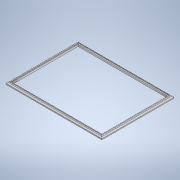
# Autodesk Inventor part: Square
Saved by Autodesk Inventor 2021 (Build 250183000, 183)
## iProperties
Created: 2022-03-13
Part Number: Square
Material: Generic
Document SubType Name: Modeling
Designer: stefi
Density: 1 g/cm^3
Appearance: Default
Author: stefi
Autodesk Inventor part; units mm, degrees
ref_plane "YZ Plane" through (0, 0, 0) normal (1, 0, 0) x (0, 1, 0)
ref_plane "XZ Plane" through (0, 0, 0) normal (0, 1, 0) x (-1, 0, 0)
ref_plane "XY Plane" through (0, 0, 0) normal (0, 0, 1) x (1, 0, 0)
sketch "Sketch2" plane through (0, 0, 0) normal (0, 1, 0) x (-1, 0, 0)
  line L0 (357.886, 268.986) -> (-357.886, 268.986)
  line L1 (-357.886, 268.986) -> (-357.886, -268.986)
  line L2 (-357.886, -268.986) -> (357.886, -268.986)
  line L3 (357.886, -268.986) -> (357.886, 268.986)
  line L4 (357.886, 268.986) -> (-357.886, -268.986) construction
  line L5 (-357.886, 268.986) -> (357.886, -268.986) construction
  line L6 (334.899, 245.999) -> (-334.899, 245.999)
  line L7 (-334.899, 245.999) -> (-334.899, -245.999)
  line L8 (-334.899, -245.999) -> (334.899, -245.999)
  line L9 (334.899, -245.999) -> (334.899, 245.999)
  line L10 (334.899, 245.999) -> (-334.899, -245.999) construction
  line L11 (-334.899, 245.999) -> (334.899, -245.999) construction
  point P0 (0, 0)
  dimension "d4" = 715.772
  dimension "d5" = 537.972
  dimension "d6" = 669.798
  dimension "d7" = 491.998
  constraints: 24 end point, 4 midpoint, 4 parallel, 2 horizontal, 2 perpendicular
  measures "d4" distance of L2.end L1.end
  measures "d5" distance of L1.end L0.end
  measures "d6" distance of L8.end L7.end
  measures "d7" distance of L7.end L6.end
extrude "Extrusion2" add sketch "Sketch2" along normal blind 13.97
fillet "Fillet1" radius 7.62 4 edges at (0, 13.97, 268.986) (357.886, 13.97, 0) (0, 13.97, -268.986) (-357.886, 13.97, 0)
sketch "Sketch3" plane through (0, 13.97, 0) normal (0, 1, 0) x (1, 0, 0)
  line L0 (350.266, 261.366) -> (350.266, -261.366) projected
  line L1 (-350.266, -261.366) -> (350.266, -261.366)
  line L2 (350.266, -261.366) -> (350.266, 261.366)
  line L3 (350.266, 261.366) -> (-350.266, 261.366)
  line L4 (-350.266, 261.366) -> (-350.266, -261.366)
  line L5 (-350.266, -261.366) -> (350.266, 261.366) construction
  line L6 (350.266, -261.366) -> (-350.266, 261.366) construction
  line L7 (-339.6244, -253.4253) -> (339.6244, -253.4253)
  line L8 (339.6244, -253.4253) -> (339.6244, 253.4253)
  line L9 (339.6244, 253.4253) -> (-339.6244, 253.4253)
  line L10 (-339.6244, 253.4253) -> (-339.6244, -253.4253)
  line L11 (-339.6244, -253.4253) -> (339.6244, 253.4253) construction
  line L12 (339.6244, -253.4253) -> (-339.6244, 253.4253) construction
  point P0 (0, 0)
  constraints: 24 end point, 4 midpoint, 4 parallel, 2 horizontal, 2 perpendicular, 1 point on line
extrude "Extrusion3" add sketch "Sketch3" along normal blind 3.81
fillet "Fillet2" radius 4.445 4 edges at (0, 17.78, 261.366) (350.266, 17.78, 0) (0, 17.78, -261.366) (-350.266, 17.78, 0)
body "Solid2"
